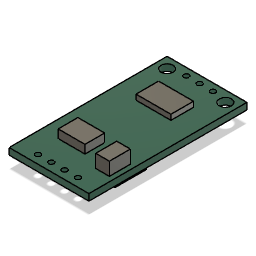
r46ca01 ds18b20 modbus (Autodesk Fusion 360 design; units mm, degrees)
Autodesk Fusion 360 part; units mm, degrees
sketch "pcb-base" plane through (0, 0, 0) normal (0, 1, 0) x (1, 0, 0)
  line L0 (7.6, -15.05) -> (-7.6, -15.05)
  line L1 (-7.6, -15.05) -> (-7.6, 15.05)
  line L2 (-7.6, 15.05) -> (7.6, 15.05)
  line L3 (7.6, 15.05) -> (7.6, -15.05)
  line L4 (7.6, -15.05) -> (-7.6, 15.05) construction
  line L5 (-7.6, -15.05) -> (7.6, 15.05) construction
  dimension "d1" = 15.2
  dimension "d2" = 30.1
  constraint horizontal L0
  constraint perpendicular L0 L1
  constraint parallel L0 L2
  constraint parallel L1 L3
  constraint coincident L4 origin
  constraint coincident L5 origin
  measures "d1" distance of L1.end L2.end
  measures "d2" distance of L0.end L1.end
extrude "Extrude1" add sketch "pcb-base" along normal blind 1.25 makes body 1
sketch "pcb-feat-mount-holes" plane through (0, 1.25, 0) normal (0, 1, 0) x (-1, 0, 0)
  line L0 (-7.6, -15.05) -> (7.6, -15.05)
  line L1 (7.6, -15.05) -> (7.6, 15.05)
  line L2 (7.6, 15.05) -> (-7.6, 15.05)
  line L3 (-7.6, 15.05) -> (-7.6, -15.05)
  circle A0 centre (5.55, -13) radius 1.15
  line L4 (0, 0) -> (0, -15.05) construction
  line L5 (0, 0) -> (7.6, 0) construction
  circle A1 centre (-5.55, -13) radius 1.15
  dimension "d5" = 2.3
  dimension "d6" = 0.9
  dimension "d7" = 0.9
  constraint coincident L4.start L5.start
  constraint midpoint L0 L4.end
  constraint midpoint L1 L5.end
  constraint symmetric A0 L4 A1
  measures "d5" diameter of A0
  measures "d6" distance of L0 A0
  measures "d7" distance of L1 A0
extrude "Extrude2" cut sketch "pcb-feat-mount-holes" against normal blind 1.25 contours A0 | A1 bodies 1
sketch "pcb-feat-terminals" plane through (0, 1.25, 0) normal (0, 1, 0) x (-1, 0, 0)
  circle A0 centre (5.55, -13) radius 1.15
  circle A1 centre (-5.55, -13) radius 1.15
  line L0 (-7.6, -15.05) -> (7.6, -15.05)
  line L1 (7.6, -15.05) -> (7.6, 15.05)
  line L2 (7.6, 15.05) -> (-7.6, 15.05)
  line L3 (-7.6, 15.05) -> (-7.6, -15.05)
  line L4 (2.54, -13.65) -> (-2.54, -13.65) construction
  circle A2 centre (2.54, -13.65) radius 0.5
  circle A3 centre (0, -13.65) radius 0.5
  circle A4 centre (-2.54, -13.65) radius 0.5
  line L5 (0, -15.05) -> (0, -11.6799) construction
  line L6 (7.6, 13.45) -> (-7.6, 13.45) construction
  circle A5 centre (3.7, 13.45) radius 0.5
  circle A6 centre (1.16, 13.45) radius 0.5
  circle A7 centre (-1.38, 13.45) radius 0.5
  circle A8 centre (-3.92, 13.45) radius 0.5
  dimension "d10" = 1
  dimension "d11" = 1
  dimension "d12" = 2.54
  dimension "d14" = 1
  dimension "d16" = 2.54
  dimension "d17" = 0.9
  dimension "d18" = 1
  dimension "d19" = 1.1
  dimension "d20" = 3.4
  dimension "d21" = 1
  dimension "d22" = 1
  dimension "d23" = 1
  dimension "d24" = 2.54
  dimension "d25" = 2.54
  dimension "d26" = 2.54
  constraint horizontal L4
  constraint coincident L4 A2.centre
  constraint coincident L4 A3.centre
  constraint coincident L4 A4.centre
  constraint midpoint L0 L5.start
  constraint perpendicular L4 L5
  constraint coincident A3.centre L5
  constraint coincident L4.end A4.centre
  constraint coincident L4.start A2.centre
  constraint coincident L1 L6.start
  constraint coincident L3 L6.end
  constraint perpendicular L3 L6
  constraint coincident L6 A5.centre
  constraint coincident L6 A6.centre
  constraint coincident L6 A7.centre
  constraint coincident L6 A8.centre
  measures "d10" diameter of A2
  measures "d11" diameter of A3
  measures "d12" distance of L4.start A3.centre
  measures "d14" diameter of A4
  measures "d16" distance of A3.centre L4.end
  measures "d17" distance of L0 A3
  measures "d18" diameter of A5
  measures "d19" distance of L2 A5
  measures "d20" distance of L6.start A5
  measures "d21" diameter of A6
  measures "d22" diameter of A7
  measures "d23" diameter of A8
  measures "d24" distance of A5.centre A6.centre
  measures "d25" distance of A6.centre A7.centre
  measures "d26" distance of A7.centre A8.centre
extrude "Extrude3" cut sketch "pcb-feat-terminals" against normal blind 1.25 contours A2 | A3 | A4 | A5 | A6 | A7 | A8 bodies 1
sketch "pcb-feat-mcu" plane through (0, 1.25, 0) normal (0, 1, 0) x (-1, 0, 0)
  circle A0 centre (1.16, 13.45) radius 0.5
  circle A1 centre (2.54, -13.65) radius 0.5
  circle A2 centre (3.7, 13.45) radius 0.5
  circle A3 centre (-1.38, 13.45) radius 0.5
  circle A4 centre (0, -13.65) radius 0.5
  circle A5 centre (-2.54, -13.65) radius 0.5
  circle A6 centre (-3.92, 13.45) radius 0.5
  circle A7 centre (5.55, -13) radius 1.15
  circle A8 centre (-5.55, -13) radius 1.15
  line L0 (-7.6, -15.05) -> (7.6, -15.05)
  line L1 (7.6, -15.05) -> (7.6, 15.05)
  line L2 (7.6, 15.05) -> (-7.6, 15.05)
  line L3 (-7.6, 15.05) -> (-7.6, -15.05)
  line L4 (-3.325, -4.85) -> (3.325, -4.85)
  line L5 (3.325, -4.85) -> (3.325, -9.15)
  line L6 (3.325, -9.15) -> (-3.325, -9.15)
  line L7 (-3.325, -9.15) -> (-3.325, -4.85)
  line L8 (-3.325, -4.85) -> (3.325, -9.15) construction
  line L9 (3.325, -4.85) -> (-3.325, -9.15) construction
  line L10 (0, -15.05) -> (0, 0) construction
  point P0 (0, -7)
  dimension "d29" = 6.65
  dimension "d30" = 4.3
  dimension "d31" = 5.9
  constraint horizontal L4
  constraint perpendicular L4 L5
  constraint parallel L4 L6
  constraint parallel L5 L7
  constraint coincident L8 P0
  constraint coincident L9 P0
  constraint midpoint L0 L10.start
  constraint coincident L10.end origin
  constraint coincident P0 L10
  measures "d29" distance of L5.end L6.end
  measures "d30" distance of L4.end L5.end
  measures "d31" distance of L0 L6
extrude "Extrude1'" add sketch "pcb-feat-mcu" along normal blind 1 separate body contours L4 L5 L6 L7 makes body 2 in component "Component"
sketch "pcb-feat-mcu-2" plane through (0, 1.25, 0) normal (0, 1, 0) x (-1, 0, 0)
  circle A0 centre (1.16, 13.45) radius 0.5
  circle A1 centre (2.54, -13.65) radius 0.5
  circle A2 centre (3.7, 13.45) radius 0.5
  circle A3 centre (-1.38, 13.45) radius 0.5
  circle A4 centre (0, -13.65) radius 0.5
  circle A5 centre (-2.54, -13.65) radius 0.5
  circle A6 centre (-3.92, 13.45) radius 0.5
  circle A7 centre (5.55, -13) radius 1.15
  circle A8 centre (-5.55, -13) radius 1.15
  line L0 (-7.6, -15.05) -> (7.6, -15.05)
  line L1 (7.6, -15.05) -> (7.6, 15.05)
  line L2 (7.6, 15.05) -> (-7.6, 15.05)
  line L3 (-7.6, 15.05) -> (-7.6, -15.05)
  line L4 (-0.7, 8.9) -> (4.4, 8.9)
  line L5 (4.4, 8.9) -> (4.4, 5.15)
  line L6 (4.4, 5.15) -> (-0.7, 5.15)
  line L7 (-0.7, 5.15) -> (-0.7, 8.9)
  line L8 (-0.7, 8.9) -> (4.4, 5.15) construction
  line L9 (4.4, 8.9) -> (-0.7, 5.15) construction
  point P0 (1.85, 7.025)
  dimension "d34" = 5.1
  dimension "d35" = 3.75
  dimension "d36" = 3.2
  dimension "d37" = 6.15
  constraint horizontal L4
  constraint perpendicular L4 L5
  constraint parallel L4 L6
  constraint parallel L5 L7
  constraint coincident L8 P0
  constraint coincident L9 P0
  measures "d34" distance of L5.end L6.end
  measures "d35" distance of L4.end L5.end
  measures "d36" distance of L1 L5
  measures "d37" distance of L2 L4
extrude "Extrude4" add sketch "pcb-feat-mcu-2" along normal blind 1.6 separate body contours L4 L5 L6 L7 makes body 3
sketch "pcb-feat-diode" plane through (0, 1.25, 0) normal (0, 1, 0) x (-1, 0, 0)
  circle A0 centre (1.16, 13.45) radius 0.5
  circle A1 centre (2.54, -13.65) radius 0.5
  circle A2 centre (3.7, 13.45) radius 0.5
  circle A3 centre (-1.38, 13.45) radius 0.5
  circle A4 centre (0, -13.65) radius 0.5
  circle A5 centre (-2.54, -13.65) radius 0.5
  circle A6 centre (-3.92, 13.45) radius 0.5
  circle A7 centre (5.55, -13) radius 1.15
  circle A8 centre (-5.55, -13) radius 1.15
  line L0 (-7.6, -15.05) -> (7.6, -15.05)
  line L1 (7.6, -15.05) -> (7.6, 15.05)
  line L2 (7.6, 15.05) -> (-7.6, 15.05)
  line L3 (-7.6, 15.05) -> (-7.6, -15.05)
  line L4 (-6.7, 10.25) -> (-4.1, 10.25)
  line L5 (-4.1, 10.25) -> (-4.1, 6.25)
  line L6 (-4.1, 6.25) -> (-6.7, 6.25)
  line L7 (-6.7, 6.25) -> (-6.7, 10.25)
  line L8 (-6.7, 10.25) -> (-4.1, 6.25) construction
  line L9 (-4.1, 10.25) -> (-6.7, 6.25) construction
  point P0 (-5.4, 8.25)
  dimension "d40" = 2.6
  dimension "d41" = 4
  dimension "d42" = 0.9
  dimension "d43" = 4.8
  constraint horizontal L4
  constraint perpendicular L4 L5
  constraint parallel L4 L6
  constraint parallel L5 L7
  constraint coincident L8 P0
  constraint coincident L9 P0
  measures "d40" distance of L5.end L6.end
  measures "d41" distance of L4.end L5.end
  measures "d42" distance of L3 L7
  measures "d43" distance of L2 L4
extrude "Extrude5" add sketch "pcb-feat-diode" along normal blind 2.5 separate body contours L4 L5 L6 L7 makes body 4
sketch "pcb-feat-vdd-reg" plane through (0, 0, 0) normal (0, -1, 0) x (1, 0, 0)
  circle A0 centre (-1.16, 13.45) radius 0.5
  circle A1 centre (-2.54, -13.65) radius 0.5
  circle A2 centre (-3.7, 13.45) radius 0.5
  circle A3 centre (1.38, 13.45) radius 0.5
  circle A4 centre (0, -13.65) radius 0.5
  circle A5 centre (2.54, -13.65) radius 0.5
  circle A6 centre (3.92, 13.45) radius 0.5
  circle A7 centre (-5.55, -13) radius 1.15
  circle A8 centre (5.55, -13) radius 1.15
  line L0 (-7.6, -15.05) -> (7.6, -15.05)
  line L1 (7.6, -15.05) -> (7.6, 15.05)
  line L2 (7.6, 15.05) -> (-7.6, 15.05)
  line L3 (-7.6, 15.05) -> (-7.6, -15.05)
  line L4 (-1, 8.1) -> (5.6, 8.1)
  line L5 (5.6, 8.1) -> (5.6, 2.1)
  line L6 (5.6, 2.1) -> (-1, 2.1)
  line L7 (-1, 2.1) -> (-1, 8.1)
  line L8 (-1, 8.1) -> (5.6, 2.1) construction
  line L9 (5.6, 8.1) -> (-1, 2.1) construction
  point P0 (2.3, 5.1)
  dimension "d46" = 6.6
  dimension "d47" = 6
  dimension "d48" = 2
  dimension "d49" = 6.95
  constraint horizontal L4
  constraint perpendicular L4 L5
  constraint parallel L4 L6
  constraint parallel L5 L7
  constraint coincident L8 P0
  constraint coincident L9 P0
  measures "d46" distance of L5.end L6.end
  measures "d47" distance of L4.end L5.end
  measures "d48" distance of L1 L5
  measures "d49" distance of L2 L4
extrude "Extrude6" add sketch "pcb-feat-vdd-reg" along normal blind 2.25 separate body contours L4 L5 L6 L7 makes body 5
component "Component" placed x (1, 0, 0) y (0, 1, 0) z (0, 0, 1) at (0, 0, 0)
equation "d6 = d7"
equation "d11 = d10"
equation "d14 = d11"
equation "d16 = d12"
equation "d18 = d10"
equation "d21 = d10"
equation "d22 = d10"
equation "d23 = d10"
equation "d24 = d12"
equation "d25 = d12"
equation "d26 = d12"
named bodies: "pcb", "mcu2", "diode", "vdd-reg"
